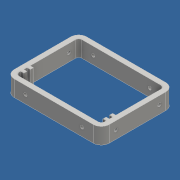
# Autodesk Inventor part: Board_holder
Saved by Autodesk Inventor 2016 (Build 200138000, 138)
## iProperties
Created: 2016-04-04
Part Number: Board_holder
Material: Generic
Document SubType Name: Modeling
Designer: admin
Density: 1 g/cm^3
Appearance: Default
Author: admin
Autodesk Inventor part; units mm, degrees
ref_plane "YZ Plane" through (0, 0, 0) normal (1, 0, 0) x (0, 1, 0)
ref_plane "XZ Plane" through (0, 0, 0) normal (0, 1, 0) x (-1, 0, 0)
ref_plane "XY Plane" through (0, 0, 0) normal (0, 0, 1) x (1, 0, 0)
sketch "Sketch1" plane through (0, 0, 0) normal (0, 0, 1) x (1, 0, 0)
  line L0 (-24.5, 22.5) -> (24.5, 22.5)
  line L1 (29.5, 17.5) -> (29.5, -17.5)
  line L2 (24.5, -22.5) -> (-24.5, -22.5)
  line L3 (-29.5, -17.5) -> (-29.5, 17.5)
  arc A0 (-24.5, 22.5) -> (-29.5, 17.5) centre (-24.5, 17.5) ccw
  arc A1 (29.5, 17.5) -> (24.5, 22.5) centre (24.5, 17.5) ccw
  arc A2 (24.5, -22.5) -> (29.5, -17.5) centre (24.5, -17.5) ccw
  arc A3 (-29.5, -17.5) -> (-24.5, -22.5) centre (-24.5, -17.5) ccw
  line L4 (-24.5, 19.5) -> (24.5, 19.5)
  line L5 (24.5, -19.5) -> (-24.5, -19.5)
  arc A4 (-24.5, 19.5) -> (-26.5, 17.5) centre (-24.5, 17.5) ccw
  arc A5 (-26.5, -17.5) -> (-24.5, -19.5) centre (-24.5, -17.5) ccw
  arc A6 (26.5, 17.5) -> (24.5, 19.5) centre (24.5, 17.5) ccw
  arc A7 (24.5, -19.5) -> (26.5, -17.5) centre (24.5, -17.5) ccw
  line L6 (-26.5, -16.5) -> (-24.5, -16.5)
  line L7 (-24.5, -16.5) -> (-24.5, -14.5)
  line L8 (-24.5, -14.5) -> (-26.5, -14.5)
  line L9 (-26.5, -12.5) -> (-24.5, -12.5)
  line L10 (-24.5, -12.5) -> (-24.5, -10.5)
  line L11 (-24.5, -10.5) -> (-26.5, -10.5)
  line L12 (26.5, -16.5) -> (24.5, -16.5)
  line L13 (24.5, -14.5) -> (26.5, -14.5)
  line L14 (26.5, -12.5) -> (24.5, -12.5)
  line L15 (24.5, -10.5) -> (26.5, -10.5)
  line L16 (-26.5, -10.5) -> (-26.5, 17.5)
  line L17 (-26.5, -17.5) -> (-26.5, -16.5)
  line L18 (-26.5, -14.5) -> (-26.5, -12.5)
  line L19 (26.5, 17.5) -> (26.5, -10.5)
  line L20 (26.5, -12.5) -> (26.5, -14.5)
  line L21 (26.5, -16.5) -> (26.5, -17.5)
  line L22 (24.5, -12.5) -> (24.5, -10.5)
  line L23 (24.5, -16.5) -> (24.5, -14.5)
  point P0 (0, 0)
  point P1 (0, 22.5)
  point P2 (-29.5, 0)
  point P3 (0, 19.5)
  point P4 (-26.5, 0)
  dimension "d0" = 5
  dimension "d1" = 59
  dimension "d2" = 45
  dimension "d4" = 3
  dimension "d6" = 3
  dimension "d7" = 2
  dimension "d8" = 2
  dimension "d9" = 3
  constraints: 48 end point, 24 tangent, 16 point on circle, 13 parallel, 11 perpendicular, 11 point on line, 8 centre point, 6 equal radius, 3 equal length, 3 horizontal, 3 midpoint, 2 collinear, 2 horizontal alignment, 2 vertical alignment, 1 coincident, 1 vertical
  measures "d0" radius of A0
  measures "d1" distance between parallel lines of L1 L3
  measures "d2" distance between parallel lines of L2 L0
  measures "d4" distance between parallel lines of L0 L4
  measures "d6" distance between parallel lines of L2 L5
  measures "d7" distance between parallel lines of L10 L16
  measures "d8" distance between parallel lines of L8 L9
  measures "d9" distance between parallel lines of L5 L6
extrude "Extrusion1" add sketch "Sketch1" along normal blind 10
sketch "Sketch3" plane through (-29.5, -17.5, 0) normal (-1, 0, 0) x (0, 0, 1)
  line L0 (0, 0) -> (0, 35) projected
  line L1 (0, 0) -> (10, 0) projected
  line L2 (10, 35) -> (10, 0) projected
  line L3 (0, 35) -> (10, 35) projected
  line L4 (5, 31) -> (5, 4) construction
  point P0 (0, 17.5)
  point P1 (5, 35)
  point P2 (0, 17.5)
  point P3 (5, 17.5)
  dimension "d20" = 27
  constraints: 3 midpoint, 2 end point, 2 vertical alignment, 1 horizontal alignment, 1 vertical
  measures "d20" distance of L4.end L4.start
sketch "Sketch2" plane through (-24.5, 22.5, 0) normal (0, 1, 0) x (1, 0, 0)
  line L0 (0, 0) -> (49, 0) projected
  line L1 (0, 0) -> (0, -10) projected
  line L2 (49, -10) -> (0, -10) projected
  line L3 (49, 0) -> (49, -10) projected
  line L4 (7, -5) -> (42, -5) construction
  point P0 (24.5, 0)
  point P1 (0, -5)
  point P2 (24.5, 0)
  point P3 (24.5, -5)
  dimension "d12" = 35
  constraints: 3 midpoint, 2 end point, 2 horizontal alignment, 1 horizontal, 1 vertical alignment
  measures "d12" distance of L4.end L4.start
hole "Hole1" at (-17.5, 22.5, 5) at (17.5, 22.5, 5) direction (0, -1, 0) diameter 2 end through all
hole "Hole2" at (-29.5, 13.5, 5) at (-29.5, -13.5, 5) direction (1, 0, 0) diameter 2 end through all
equation "\"d4\" = d3"
equation "\"d6\" = d3"
equation "\"d3\" = 3"
body "Solid1"
